Autodesk Fusion 360 part; units mm, degrees
(part 2 of 3)
  dimension "d109" = 3.1
  dimension "d110" = 3.1
  dimension "d111" = 3.1
  dimension "d112" = 3.1
  constraint parallel L339 L340
  constraint parallel L341 L342
  constraint tangent A29 L348
  constraint perpendicular L59 L347
  constraint perpendicular L59 L349
  constraint parallel L347 L348
  constraint parallel L10 L349
  constraint tangent A344 L353
  constraint tangent A347 L353
  constraint tangent L352 A347
  constraint tangent A344 L350
  constraint tangent A346 L352
  constraint tangent L350 A345
  constraint tangent L351 A346
  constraint tangent A345 L351
  constraint coincident P12 A348.centre
  constraint coincident P13 A349.centre
  constraint coincident P0 A350.centre
  constraint coincident P1 A351.centre
  constraint coincident P2 A352.centre
  constraint coincident P3 A353.centre
  constraint coincident P4 A354.centre
  constraint coincident P5 A355.centre
  constraint coincident P6 A356.centre
  constraint coincident P7 A357.centre
  constraint coincident P8 A358.centre
  constraint coincident P9 A359.centre
  constraint coincident P10 A360.centre
  constraint coincident P11 A361.centre
  constraint tangent L344 A341
  constraint tangent L343 A343
  constraint tangent L345 A342
  constraint tangent A341 L345
  constraint tangent L343 A340
  constraint tangent A340 L344
  constraint tangent A342 L346
  constraint tangent L346 A343
  measures "d99" diameter of A348
  measures "d100" diameter of A349
  measures "d101" diameter of A350
  measures "d102" diameter of A351
  measures "d103" diameter of A352
  measures "d104" diameter of A353
  measures "d105" diameter of A354
  measures "d106" diameter of A355
  measures "d107" diameter of A356
  measures "d108" diameter of A357
  measures "d109" diameter of A358
  measures "d110" diameter of A359
  measures "d111" diameter of A360
  measures "d112" diameter of A361
ref_plane "WorkPlane1" through (183.3563, -53.8188, -3) normal (0, 0, 1) x (1, 0, 0)
sketch "Sketch2" plane through (183.3563, -53.8188, -3) normal (0, 0, 1) x (1, 0, 0)
  line L0 (180.9997, -53.2885) -> (-181.0002, -53.2885)
  arc A0 (-185.0002, -49.2885) -> (-181.0002, -53.2885) centre (-181.0002, -49.2885) ccw
  line L1 (-185.0002, -49.2885) -> (-185.0002, 48.7115)
  arc A1 (-181.0002, 52.7115) -> (-185.0002, 48.7115) centre (-181.0002, 48.7115) ccw
  line L2 (-181.0002, 52.7115) -> (-28.9625, 52.7115)
  line L3 (-28.9625, 52.7115) -> (-28.9625, 55.9115)
  line L4 (-13.9625, 55.9115) -> (-13.9625, 52.7115)
  line L5 (-13.9625, 52.7115) -> (180.9997, 52.7115)
  arc A2 (184.9997, 48.7115) -> (180.9997, 52.7115) centre (180.9997, 48.7115) ccw
  line L6 (184.9997, 48.7115) -> (184.9997, -49.2885)
  arc A3 (180.9997, -53.2885) -> (184.9997, -49.2885) centre (180.9997, -49.2885) ccw
  line L7 (-13.9625, 55.9115) -> (-13.9625, 59.7113)
  line L8 (-28.9625, 55.9115) -> (-28.9625, 59.7113)
  arc A4 (196.0613, 54.7113) -> (188.0613, 62.7113) centre (188.0613, 54.7113) ccw
  line L9 (-13.9625, 62.7113) -> (188.0613, 62.7113)
  line L10 (-188.0613, 62.7113) -> (-28.9625, 62.7113)
  arc A5 (-188.0613, 62.7113) -> (-196.0613, 54.7113) centre (-188.0613, 54.7113) ccw
  line L11 (-196.0613, -54.7113) -> (-196.0613, 54.7113)
  arc A6 (-196.0613, -54.7113) -> (-188.0613, -62.7112) centre (-188.0613, -54.7113) ccw
  line L12 (188.0613, -62.7112) -> (-188.0613, -62.7112)
  arc A7 (188.0613, -62.7112) -> (196.0613, -54.7113) centre (188.0613, -54.7113) ccw
  line L13 (196.0612, 54.7113) -> (196.0612, -54.7113)
  line L14 (-28.9625, 59.7113) -> (-28.9625, 62.7113)
  line L15 (-13.9625, 59.7113) -> (-13.9625, 62.7113)
  line L16 (-61.8591, 54.9113) -> (-60.5312, 57.2113)
  line L17 (-60.5312, 57.2113) -> (-61.8591, 59.5113)
  line L18 (-61.8591, 59.5113) -> (-64.5149, 59.5113)
  line L19 (-64.5149, 59.5113) -> (-65.8428, 57.2113)
  line L20 (-65.8428, 57.2113) -> (-64.5149, 54.9113)
  line L21 (-64.5149, 54.9113) -> (-61.8591, 54.9113)
  line L22 (-125.0463, 54.9113) -> (-123.7184, 57.2113)
  line L23 (-123.7184, 57.2113) -> (-125.0463, 59.5113)
  line L24 (-125.0463, 59.5113) -> (-127.7022, 59.5113)
  line L25 (-127.7022, 59.5113) -> (-129.0301, 57.2113)
  line L26 (-129.0301, 57.2113) -> (-127.7022, 54.9113)
  line L27 (-127.7022, 54.9113) -> (-125.0463, 54.9113)
  line L28 (-188.2613, 29.4334) -> (-190.5613, 30.7613)
  line L29 (-190.5613, 30.7613) -> (-192.8613, 29.4334)
  line L30 (-192.8613, 29.4334) -> (-192.8613, 26.7776)
  line L31 (-192.8613, 26.7776) -> (-190.5613, 25.4497)
  line L32 (-190.5613, 25.4497) -> (-188.2613, 26.7776)
  line L33 (-188.2613, 26.7776) -> (-188.2613, 29.4334)
  line L34 (-188.2613, -26.7776) -> (-190.5613, -25.4497)
  line L35 (-190.5613, -25.4497) -> (-192.8613, -26.7776)
  line L36 (-192.8613, -26.7776) -> (-192.8613, -29.4334)
  line L37 (-192.8613, -29.4334) -> (-190.5613, -30.7613)
  line L38 (-190.5613, -30.7613) -> (-188.2613, -29.4334)
  line L39 (-188.2613, -29.4334) -> (-188.2613, -26.7776)
  line L40 (-127.7022, -54.9112) -> (-129.0301, -57.2112)
  line L41 (-129.0301, -57.2112) -> (-127.7022, -59.5112)
  line L42 (-127.7022, -59.5112) -> (-125.0463, -59.5112)
  line L43 (-125.0463, -59.5112) -> (-123.7184, -57.2112)
  line L44 (-123.7184, -57.2112) -> (-125.0463, -54.9112)
  line L45 (-125.0463, -54.9112) -> (-127.7022, -54.9112)
  line L46 (-64.5149, -54.9112) -> (-65.8428, -57.2112)
  line L47 (-65.8428, -57.2112) -> (-64.5149, -59.5112)
  line L48 (-64.5149, -59.5112) -> (-61.8591, -59.5112)
  line L49 (-61.8591, -59.5112) -> (-60.5312, -57.2112)
  line L50 (-60.5312, -57.2112) -> (-61.8591, -54.9112)
  line L51 (-61.8591, -54.9112) -> (-64.5149, -54.9112)
  line L52 (-1.3282, -54.9114) -> (-2.6558, -57.2116)
  line L53 (-2.6558, -57.2116) -> (-1.3276, -59.5114)
  line L54 (-1.3276, -59.5114) -> (1.3282, -59.5111)
  line L55 (1.3282, -59.5111) -> (2.6558, -57.2109)
  line L56 (2.6558, -57.2109) -> (1.3276, -54.9111)
  line L57 (1.3276, -54.9111) -> (-1.3282, -54.9114)
  line L58 (61.8591, -54.9112) -> (60.5312, -57.2112)
  line L59 (60.5312, -57.2112) -> (61.8591, -59.5112)
  line L60 (61.8591, -59.5112) -> (64.5149, -59.5112)
  line L61 (64.5149, -59.5112) -> (65.8428, -57.2112)
  line L62 (65.8428, -57.2112) -> (64.5149, -54.9112)
  line L63 (64.5149, -54.9112) -> (61.8591, -54.9112)
  line L64 (125.0463, -54.9112) -> (123.7184, -57.2112)
  line L65 (123.7184, -57.2112) -> (125.0463, -59.5112)
  line L66 (125.0463, -59.5112) -> (127.7022, -59.5112)
  line L67 (127.7022, -59.5112) -> (129.0301, -57.2112)
  line L68 (129.0301, -57.2112) -> (127.7022, -54.9112)
  line L69 (127.7022, -54.9112) -> (125.0463, -54.9112)
  line L70 (188.2612, -29.4334) -> (190.5612, -30.7613)
  line L71 (190.5612, -30.7613) -> (192.8612, -29.4334)
  line L72 (192.8612, -29.4334) -> (192.8612, -26.7776)
  line L73 (192.8612, -26.7776) -> (190.5612, -25.4497)
  line L74 (190.5612, -25.4497) -> (188.2612, -26.7776)
  line L75 (188.2612, -26.7776) -> (188.2612, -29.4334)
  line L76 (188.2612, 26.7776) -> (190.5612, 25.4497)
  line L77 (190.5612, 25.4497) -> (192.8612, 26.7776)
  line L78 (192.8612, 26.7776) -> (192.8612, 29.4334)
  line L79 (192.8612, 29.4334) -> (190.5612, 30.7613)
  line L80 (190.5612, 30.7613) -> (188.2612, 29.4334)
  line L81 (188.2612, 29.4334) -> (188.2612, 26.7776)
  line L82 (127.7022, 54.9113) -> (129.0301, 57.2113)
  line L83 (129.0301, 57.2113) -> (127.7022, 59.5113)
  line L84 (127.7022, 59.5113) -> (125.0463, 59.5113)
  line L85 (125.0463, 59.5113) -> (123.7184, 57.2113)
  line L86 (123.7184, 57.2113) -> (125.0463, 54.9113)
  line L87 (125.0463, 54.9113) -> (127.7022, 54.9113)
  line L88 (64.5149, 54.9113) -> (65.8428, 57.2113)
  line L89 (65.8428, 57.2113) -> (64.5149, 59.5113)
  line L90 (64.5149, 59.5113) -> (61.8591, 59.5113)
  line L91 (61.8591, 59.5113) -> (60.5312, 57.2113)
  line L92 (60.5312, 57.2113) -> (61.8591, 54.9113)
  line L93 (61.8591, 54.9113) -> (64.5149, 54.9113)
  line L94 (1.3279, 54.9113) -> (2.6558, 57.2113)
  line L95 (2.6558, 57.2113) -> (1.3279, 59.5113)
  line L96 (1.3279, 59.5113) -> (-1.3279, 59.5113)
  line L97 (-1.3279, 59.5113) -> (-2.6558, 57.2113)
  line L98 (-2.6558, 57.2113) -> (-1.3279, 54.9113)
  line L99 (-1.3279, 54.9113) -> (1.3279, 54.9113)
  point P0 (-126.3743, 57.2113)
  point P1 (-190.5613, 28.1055)
  point P2 (-190.5613, -28.1055)
  point P3 (-126.3743, -57.2112)
  point P4 (-63.187, -57.2112)
  point P5 (0, -57.2112)
  point P6 (63.187, -57.2112)
  point P7 (126.3742, -57.2112)
  point P8 (190.5612, -28.1055)
  point P9 (190.5612, 28.1055)
  point P10 (126.3742, 57.2113)
  point P11 (63.187, 57.2113)
  point P12 (0, 57.2113)
  point P13 (-63.187, 57.2113)
  point P14 (0, 57.2113)
  point P15 (-63.187, 57.2113)
  point P16 (-126.3743, 57.2113)
  point P17 (-190.5613, 28.1055)
  point P18 (-190.5613, -28.1055)
  point P19 (-126.3743, -57.2112)
  point P20 (-63.187, -57.2112)
  point P21 (0, -57.2112)
  point P22 (63.187, -57.2112)
  point P23 (126.3742, -57.2112)
  point P24 (190.5612, -28.1055)
  point P25 (190.5612, 28.1055)
  point P26 (126.3742, 57.2113)
  point P27 (63.187, 57.2113)
  point P28 (-63.187, 57.2113)
  point P29 (-126.3743, 57.2113)
  point P30 (-190.5613, 28.1055)
  point P31 (-190.5613, -28.1055)
  point P32 (-126.3743, -57.2112)
  point P33 (-63.187, -57.2112)
  point P34 (0, -57.2112)
  point P35 (63.187, -57.2112)
  point P36 (126.3742, -57.2112)
  point P37 (190.5612, -28.1055)
  point P38 (190.5612, 28.1055)
  point P39 (126.3742, 57.2113)
  point P40 (63.187, 57.2113)
  point P41 (0, 57.2113)
  dimension "d113" = 2.3
  dimension "d114" = 2.3
  dimension "d115" = 2.3
  dimension "d116" = 2.3
  dimension "d117" = 2.3
  dimension "d118" = 2.3
  dimension "d119" = 2.3
  dimension "d120" = 2.3
  dimension "d121" = 2.3
  dimension "d122" = 2.3
  dimension "d123" = 2.3
  dimension "d124" = 2.3
  dimension "d125" = 2.3
  dimension "d126" = 2.3
  constraint tangent L1 A1
  constraint tangent L0 A3
  constraint tangent L0 A0
  constraint tangent A0 L1
  constraint tangent A1 L2
  constraint tangent L5 A2
  constraint tangent A2 L6
  constraint tangent L6 A3
  constraint perpendicular L10 L14
  constraint perpendicular L9 L15
  constraint tangent A4 L13
  constraint tangent A4 L9
  constraint tangent L10 A5
  constraint tangent A5 L11
  constraint tangent L11 A6
  constraint tangent A6 L12
  constraint tangent L12 A7
  constraint tangent A7 L13
  constraint coincident P41 P14
  constraint coincident P28 P15
  constraint coincident P29 P16
  constraint coincident P30 P17
  constraint coincident P31 P18
  constraint coincident P32 P19
  constraint coincident P33 P20
  constraint coincident P34 P21
  constraint coincident P35 P22
  constraint coincident P36 P23
  constraint coincident P37 P24
  constraint coincident P38 P25
  constraint coincident P39 P26
  constraint coincident P40 P27
  measures "d113" distance of P28 L21
  measures "d114" distance of P29 L27
  measures "d115" distance of P30 L33
  measures "d116" distance of P31 L39
  measures "d117" distance of P32 L45
  measures "d118" distance of P33 L51
  measures "d119" distance of P34 L57
  measures "d120" distance of P35 L63
  measures "d121" distance of P36 L69
  measures "d122" distance of P37 L75
  measures "d123" distance of P38 L81
  measures "d124" distance of P39 L87
  measures "d125" distance of P40 L93
  measures "d126" distance of P41 L99
ref_plane "WorkPlane2" through (183.3562, -53.8188, -9) normal (0, 0, 1) x (1, 0, 0)
ref_plane "WorkPlane3" through (183.3562, -53.8188, -9) normal (0, 0, 1) x (1, 0, 0)
sketch "Sketch4" plane through (183.3562, -53.8188, -9) normal (0, 0, 1) x (1, 0, 0)
  line L0 (-188.0613, 62.7113) -> (188.0613, 62.7113)
  arc A0 (-188.0613, 62.7113) -> (-196.0613, 54.7113) centre (-188.0613, 54.7113) ccw
  line L1 (-196.0613, -54.7113) -> (-196.0613, 54.7113)
  circle A1 centre (-190.5613, 28.1055) radius 1.55
  circle A2 centre (-190.5613, -28.1055) radius 1.55
  circle A3 centre (-126.3742, 57.2113) radius 1.55
  arc A4 (-196.0613, -54.7113) -> (-188.0613, -62.7113) centre (-188.0613, -54.7113) ccw
  line L2 (188.0613, -62.7113) -> (-188.0613, -62.7112)
  circle A5 centre (-126.3742, -57.2113) radius 1.55
  circle A6 centre (-63.187, -57.2113) radius 1.55
  circle A7 centre (-63.187, 57.2113) radius 1.55
  circle A8 centre (0, 57.2113) radius 1.55
  circle A9 centre (0, -57.2113) radius 1.55
  circle A10 centre (63.187, -57.2113) radius 1.55
  circle A11 centre (126.3742, -57.2113) radius 1.55
  circle A12 centre (63.187, 57.2113) radius 1.55
  circle A13 centre (126.3742, 57.2113) radius 1.55
  arc A14 (196.0612, 54.7113) -> (188.0613, 62.7112) centre (188.0613, 54.7113) ccw
  line L3 (196.0612, 54.7113) -> (196.0613, -54.7113)
  circle A15 centre (190.5613, 28.1055) radius 1.55
  circle A16 centre (190.5613, -28.1055) radius 1.55
  arc A17 (188.0613, -62.7113) -> (196.0613, -54.7113) centre (188.0613, -54.7113) ccw
  point P0 (0, -57.2113)
  point P1 (0, 57.2113)
  point P2 (126.3742, 57.2113)
extrude "Extrude8" add sketch "Frogdor Top Plate" against normal blind 3 makes body 1
extrude "Extrude9" add sketch "Sketch2" against normal blind 6 separate body makes body 2
extrude "Extrude10" add sketch "Sketch4" against normal blind 3 separate body makes body 3
sketch "Sketch5" plane through (0, 0, 0) normal (0, 0, 1) x (-1, 0, 0)
  arc A0 (-351.1875, 6.3375) -> (-350.1875, 7.3375) centre (-351.1875, 7.3375) ccw
  line L0 (-351.1875, 6.3375) -> (-363.1875, 6.3375)
  arc A1 (-364.1875, 7.3375) -> (-363.1875, 6.3375) centre (-363.1875, 7.3375) ccw
  line L1 (-364.1875, 7.3375) -> (-364.1875, 19.3375)
  arc A2 (-363.1875, 20.3375) -> (-364.1875, 19.3375) centre (-363.1875, 19.3375) ccw
  line L2 (-363.1875, 20.3375) -> (-351.1875, 20.3375)
  arc A3 (-350.1875, 19.3375) -> (-351.1875, 20.3375) centre (-351.1875, 19.3375) ccw
  line L3 (-350.1875, 19.3375) -> (-350.1875, 7.3375)
  arc A4 (-187.975, 26.3875) -> (-186.975, 25.3875) centre (-186.975, 26.3875) ccw
  line L4 (-187.975, 26.3875) -> (-187.975, 38.3875)
  arc A5 (-186.975, 39.3875) -> (-187.975, 38.3875) centre (-186.975, 38.3875) ccw
  line L5 (-186.975, 39.3875) -> (-174.975, 39.3875)
  arc A6 (-173.975, 38.3875) -> (-174.975, 39.3875) centre (-174.975, 38.3875) ccw
  line L6 (-173.975, 38.3875) -> (-173.975, 26.3875)
  arc A7 (-174.975, 25.3875) -> (-173.975, 26.3875) centre (-174.975, 26.3875) ccw
  line L7 (-174.975, 25.3875) -> (-186.975, 25.3875)
  arc A8 (-270.225, 25.3875) -> (-269.225, 26.3875) centre (-270.225, 26.3875) ccw
  line L8 (-270.225, 25.3875) -> (-282.225, 25.3875)
  arc A9 (-283.225, 26.3875) -> (-282.225, 25.3875) centre (-282.225, 26.3875) ccw
  line L9 (-283.225, 26.3875) -> (-283.225, 38.3875)
  arc A10 (-282.225, 39.3875) -> (-283.225, 38.3875) centre (-282.225, 38.3875) ccw
  line L10 (-282.225, 39.3875) -> (-270.225, 39.3875)
  arc A11 (-269.225, 38.3875) -> (-270.225, 39.3875) centre (-270.225, 38.3875) ccw
  line L11 (-269.225, 38.3875) -> (-269.225, 26.3875)
  arc A12 (-313.0875, 25.3875) -> (-312.0875, 26.3875) centre (-313.0875, 26.3875) ccw
  line L12 (-313.0875, 25.3875) -> (-325.0875, 25.3875)
  arc A13 (-326.0875, 26.3875) -> (-325.0875, 25.3875) centre (-325.0875, 26.3875) ccw
  line L13 (-326.0875, 26.3875) -> (-326.0875, 38.3875)
  arc A14 (-325.0875, 39.3875) -> (-326.0875, 38.3875) centre (-325.0875, 38.3875) ccw
  line L14 (-325.0875, 39.3875) -> (-313.0875, 39.3875)
  arc A15 (-312.0875, 38.3875) -> (-313.0875, 39.3875) centre (-313.0875, 38.3875) ccw
  line L15 (-312.0875, 38.3875) -> (-312.0875, 26.3875)
  arc A16 (-305.9438, 44.4375) -> (-304.9438, 45.4375) centre (-305.9438, 45.4375) ccw
  line L16 (-305.9438, 44.4375) -> (-317.9438, 44.4375)
  arc A17 (-318.9438, 45.4375) -> (-317.9438, 44.4375) centre (-317.9438, 45.4375) ccw
  line L17 (-318.9438, 45.4375) -> (-318.9438, 57.4375)
  arc A18 (-317.9438, 58.4375) -> (-318.9438, 57.4375) centre (-317.9438, 57.4375) ccw
  line L18 (-317.9438, 58.4375) -> (-305.9438, 58.4375)
  arc A19 (-304.9438, 57.4375) -> (-305.9438, 58.4375) centre (-305.9438, 57.4375) ccw
  line L19 (-304.9438, 57.4375) -> (-304.9438, 45.4375)
  arc A20 (-217.8375, 44.4375) -> (-216.8375, 45.4375) centre (-217.8375, 45.4375) ccw
  line L20 (-217.8375, 44.4375) -> (-229.8375, 44.4375)
  arc A21 (-230.8375, 45.4375) -> (-229.8375, 44.4375) centre (-229.8375, 45.4375) ccw
  line L21 (-230.8375, 45.4375) -> (-230.8375, 57.4375)
  arc A22 (-229.8375, 58.4375) -> (-230.8375, 57.4375) centre (-229.8375, 57.4375) ccw
  line L22 (-229.8375, 58.4375) -> (-217.8375, 58.4375)
  arc A23 (-216.8375, 57.4375) -> (-217.8375, 58.4375) centre (-217.8375, 57.4375) ccw
  line L23 (-216.8375, 57.4375) -> (-216.8375, 45.4375)
  arc A24 (-122.5875, 44.4375) -> (-121.5875, 45.4375) centre (-122.5875, 45.4375) ccw
  line L24 (-122.5875, 44.4375) -> (-134.5875, 44.4375)
  arc A25 (-135.5875, 45.4375) -> (-134.5875, 44.4375) centre (-134.5875, 45.4375) ccw
  line L25 (-135.5875, 45.4375) -> (-135.5875, 57.4375)
  arc A26 (-134.5875, 58.4375) -> (-135.5875, 57.4375) centre (-134.5875, 57.4375) ccw
  line L26 (-134.5875, 58.4375) -> (-122.5875, 58.4375)
  arc A27 (-121.5875, 57.4375) -> (-122.5875, 58.4375) centre (-122.5875, 57.4375) ccw
  line L27 (-121.5875, 57.4375) -> (-121.5875, 45.4375)
  arc A28 (-236.8875, 44.4375) -> (-235.8875, 45.4375) centre (-236.8875, 45.4375) ccw
  line L28 (-236.8875, 44.4375) -> (-248.8875, 44.4375)
  arc A29 (-249.8875, 45.4375) -> (-248.8875, 44.4375) centre (-248.8875, 45.4375) ccw
  line L29 (-249.8875, 45.4375) -> (-249.8875, 57.4375)
  arc A30 (-248.8875, 58.4375) -> (-249.8875, 57.4375) centre (-248.8875, 57.4375) ccw
  line L30 (-248.8875, 58.4375) -> (-236.8875, 58.4375)
  arc A31 (-235.8875, 57.4375) -> (-236.8875, 58.4375) centre (-236.8875, 57.4375) ccw
  line L31 (-235.8875, 57.4375) -> (-235.8875, 45.4375)
  arc A32 (-297.5057, 45.4375) -> (-296.5057, 46.4375) centre (-297.5057, 46.4375) ccw
  line L32 (-297.5057, 45.4375) -> (-302.5057, 45.4375)
  arc A33 (-303.5057, 46.4375) -> (-302.5057, 45.4375) centre (-302.5057, 46.4375) ccw
  line L33 (-303.5057, 46.4375) -> (-303.5057, 59.4375)
  arc A34 (-302.5057, 60.4375) -> (-303.5058, 59.4375) centre (-302.5058, 59.4375) ccw
  line L34 (-302.5057, 60.4375) -> (-297.5057, 60.4375)
  arc A35 (-296.5057, 59.4375) -> (-297.5057, 60.4375) centre (-297.5057, 59.4375) ccw
  line L35 (-296.5057, 59.4375) -> (-296.5057, 46.4375)
  arc A36 (-117.825, 25.3875) -> (-116.825, 26.3875) centre (-117.825, 26.3875) ccw
  line L36 (-117.825, 25.3875) -> (-129.825, 25.3875)
  arc A37 (-130.825, 26.3875) -> (-129.825, 25.3875) centre (-129.825, 26.3875) ccw
  line L37 (-130.825, 26.3875) -> (-130.825, 38.3875)
  arc A38 (-129.825, 39.3875) -> (-130.825, 38.3875) centre (-129.825, 38.3875) ccw
  line L38 (-129.825, 39.3875) -> (-117.825, 39.3875)
  arc A39 (-116.825, 38.3875) -> (-117.825, 39.3875) centre (-117.825, 38.3875) ccw
  line L39 (-116.825, 38.3875) -> (-116.825, 26.3875)
  arc A40 (-3.525, 25.3875) -> (-2.525, 26.3875) centre (-3.525, 26.3875) ccw
  line L40 (-3.525, 25.3875) -> (-15.525, 25.3875)
  arc A41 (-16.525, 26.3875) -> (-15.525, 25.3875) centre (-15.525, 26.3875) ccw
  line L41 (-16.525, 26.3875) -> (-16.525, 38.3875)
  arc A42 (-15.525, 39.3875) -> (-16.525, 38.3875) centre (-15.525, 38.3875) ccw
  line L42 (-15.525, 39.3875) -> (-3.525, 39.3875)
  arc A43 (-2.525, 38.3875) -> (-3.525, 39.3875) centre (-3.525, 38.3875) ccw
  line L43 (-2.525, 38.3875) -> (-2.525, 26.3875)
  line L44 (-83.4875, 57.4375) -> (-83.4875, 45.4375)
  arc A44 (-84.4875, 44.4375) -> (-83.4875, 45.4375) centre (-84.4875, 45.4375) ccw
  line L45 (-84.4875, 44.4375) -> (-96.4875, 44.4375)
  arc A45 (-97.4875, 45.4375) -> (-96.4875, 44.4375) centre (-96.4875, 45.4375) ccw
  line L46 (-97.4875, 45.4375) -> (-97.4875, 57.4375)
  arc A46 (-96.4875, 58.4375) -> (-97.4875, 57.4375) centre (-96.4875, 57.4375) ccw
  line L47 (-96.4875, 58.4375) -> (-84.4875, 58.4375)
  arc A47 (-83.4875, 57.4375) -> (-84.4875, 58.4375) centre (-84.4875, 57.4375) ccw
  arc A48 (-103.5375, 44.4375) -> (-102.5375, 45.4375) centre (-103.5375, 45.4375) ccw
  line L48 (-103.5375, 44.4375) -> (-115.5375, 44.4375)
  arc A49 (-116.5375, 45.4375) -> (-115.5375, 44.4375) centre (-115.5375, 45.4375) ccw
  line L49 (-116.5375, 45.4375) -> (-116.5375, 57.4375)
  arc A50 (-115.5375, 58.4375) -> (-116.5375, 57.4375) centre (-115.5375, 57.4375) ccw
  line L50 (-115.5375, 58.4375) -> (-103.5375, 58.4375)
  arc A51 (-102.5375, 57.4375) -> (-103.5375, 58.4375) centre (-103.5375, 57.4375) ccw
  line L51 (-102.5375, 57.4375) -> (-102.5375, 45.4375)
  arc A52 (-255.9375, 44.4375) -> (-254.9375, 45.4375) centre (-255.9375, 45.4375) ccw
  line L52 (-255.9375, 44.4375) -> (-267.9375, 44.4375)
  arc A53 (-268.9375, 45.4375) -> (-267.9375, 44.4375) centre (-267.9375, 45.4375) ccw
  line L53 (-268.9375, 45.4375) -> (-268.9375, 57.4375)
  arc A54 (-267.9375, 58.4375) -> (-268.9375, 57.4375) centre (-267.9375, 57.4375) ccw
  line L54 (-267.9375, 58.4375) -> (-255.9375, 58.4375)
  arc A55 (-254.9375, 57.4375) -> (-255.9375, 58.4375) centre (-255.9375, 57.4375) ccw
  line L55 (-254.9375, 57.4375) -> (-254.9375, 45.4375)
  arc A56 (-165.45, 6.3375) -> (-164.45, 7.3375) centre (-165.45, 7.3375) ccw
  line L56 (-165.45, 6.3375) -> (-177.45, 6.3375)
  arc A57 (-178.45, 7.3375) -> (-177.45, 6.3375) centre (-177.45, 7.3375) ccw
  line L57 (-178.45, 7.3375) -> (-178.45, 19.3375)
  arc A58 (-177.45, 20.3375) -> (-178.45, 19.3375) centre (-177.45, 19.3375) ccw
  line L58 (-177.45, 20.3375) -> (-165.45, 20.3375)
  arc A59 (-164.45, 19.3375) -> (-165.45, 20.3375) centre (-165.45, 19.3375) ccw
  line L59 (-164.45, 19.3375) -> (-164.45, 7.3375)
  arc A60 (-226.075, 26.3875) -> (-225.075, 25.3875) centre (-225.075, 26.3875) ccw
  line L60 (-226.075, 26.3875) -> (-226.075, 38.3875)
  arc A61 (-225.075, 39.3875) -> (-226.075, 38.3875) centre (-225.075, 38.3875) ccw
  line L61 (-225.075, 39.3875) -> (-213.075, 39.3875)
  arc A62 (-212.075, 38.3875) -> (-213.075, 39.3875) centre (-213.075, 38.3875) ccw
  line L62 (-212.075, 38.3875) -> (-212.075, 26.3875)
  arc A63 (-213.075, 25.3875) -> (-212.075, 26.3875) centre (-213.075, 26.3875) ccw
  line L63 (-213.075, 25.3875) -> (-225.075, 25.3875)
  arc A64 (-194.025, 25.3875) -> (-193.025, 26.3875) centre (-194.025, 26.3875) ccw
  line L64 (-194.025, 25.3875) -> (-206.025, 25.3875)
  arc A65 (-207.025, 26.3875) -> (-206.025, 25.3875) centre (-206.025, 26.3875) ccw
  line L65 (-207.025, 26.3875) -> (-207.025, 38.3875)
  arc A66 (-206.025, 39.3875) -> (-207.025, 38.3875) centre (-206.025, 38.3875) ccw
  line L66 (-206.025, 39.3875) -> (-194.025, 39.3875)
  arc A67 (-193.025, 38.3875) -> (-194.025, 39.3875) centre (-194.025, 38.3875) ccw
  line L67 (-193.025, 38.3875) -> (-193.025, 26.3875)
  arc A68 (-260.7, 6.3375) -> (-259.7, 7.3375) centre (-260.7, 7.3375) ccw
  line L68 (-260.7, 6.3375) -> (-272.7, 6.3375)
  arc A69 (-273.7, 7.3375) -> (-272.7, 6.3375) centre (-272.7, 7.3375) ccw
  line L69 (-273.7, 7.3375) -> (-273.7, 19.3375)
  arc A70 (-272.7, 20.3375) -> (-273.7, 19.3375) centre (-272.7, 19.3375) ccw
  line L70 (-272.7, 20.3375) -> (-260.7, 20.3375)
  arc A71 (-259.7, 19.3375) -> (-260.7, 20.3375) centre (-260.7, 19.3375) ccw
  line L71 (-259.7, 19.3375) -> (-259.7, 7.3375)
  arc A72 (-160.6875, 44.4375) -> (-159.6875, 45.4375) centre (-160.6875, 45.4375) ccw
  line L72 (-160.6875, 44.4375) -> (-172.6875, 44.4375)
  arc A73 (-173.6875, 45.4375) -> (-172.6875, 44.4375) centre (-172.6875, 45.4375) ccw
  line L73 (-173.6875, 45.4375) -> (-173.6875, 57.4375)
  arc A74 (-172.6875, 58.4375) -> (-173.6875, 57.4375) centre (-172.6875, 57.4375) ccw
  line L74 (-172.6875, 58.4375) -> (-160.6875, 58.4375)
  arc A75 (-159.6875, 57.4375) -> (-160.6875, 58.4375) centre (-160.6875, 57.4375) ccw
  line L75 (-159.6875, 57.4375) -> (-159.6875, 45.4375)
  arc A76 (-55.9125, 25.3875) -> (-54.9125, 26.3875) centre (-55.9125, 26.3875) ccw
  line L76 (-55.9125, 25.3875) -> (-67.9125, 25.3875)
  arc A77 (-68.9125, 26.3875) -> (-67.9125, 25.3875) centre (-67.9125, 26.3875) ccw
  line L77 (-68.9125, 26.3875) -> (-68.9125, 38.3875)
  arc A78 (-67.9125, 39.3875) -> (-68.9125, 38.3875) centre (-67.9125, 38.3875) ccw
  line L78 (-67.9125, 39.3875) -> (-55.9125, 39.3875)
  arc A79 (-54.9125, 38.3875) -> (-55.9125, 39.3875) centre (-55.9125, 38.3875) ccw
  line L79 (-54.9125, 38.3875) -> (-54.9125, 26.3875)
  arc A80 (-351.1875, 25.3875) -> (-350.1875, 26.3875) centre (-351.1875, 26.3875) ccw
  line L80 (-351.1875, 25.3875) -> (-363.1875, 25.3875)
  arc A81 (-364.1875, 26.3875) -> (-363.1875, 25.3875) centre (-363.1875, 26.3875) ccw
  line L81 (-364.1875, 26.3875) -> (-364.1875, 38.3875)
  arc A82 (-363.1875, 39.3875) -> (-364.1875, 38.3875) centre (-363.1875, 38.3875) ccw
  line L82 (-363.1875, 39.3875) -> (-351.1875, 39.3875)
  arc A83 (-350.1875, 38.3875) -> (-351.1875, 39.3875) centre (-351.1875, 38.3875) ccw
  line L83 (-350.1875, 38.3875) -> (-350.1875, 26.3875)
  arc A84 (-79.725, 25.3875) -> (-78.725, 26.3875) centre (-79.725, 26.3875) ccw
  line L84 (-79.725, 25.3875) -> (-91.725, 25.3875)
  arc A85 (-92.725, 26.3875) -> (-91.725, 25.3875) centre (-91.725, 26.3875) ccw
  line L85 (-92.725, 26.3875) -> (-92.725, 38.3875)
  arc A86 (-91.725, 39.3875) -> (-92.725, 38.3875) centre (-91.725, 38.3875) ccw
  line L86 (-91.725, 39.3875) -> (-79.725, 39.3875)
  arc A87 (-78.725, 38.3875) -> (-79.725, 39.3875) centre (-79.725, 38.3875) ccw
  line L87 (-78.725, 38.3875) -> (-78.725, 26.3875)
  arc A88 (-155.925, 25.3875) -> (-154.925, 26.3875) centre (-155.925, 26.3875) ccw
  line L88 (-155.925, 25.3875) -> (-167.925, 25.3875)
  arc A89 (-168.925, 26.3875) -> (-167.925, 25.3875) centre (-167.925, 26.3875) ccw
  line L89 (-168.925, 26.3875) -> (-168.925, 38.3875)
  arc A90 (-167.925, 39.3875) -> (-168.925, 38.3875) centre (-167.925, 38.3875) ccw
  line L90 (-167.925, 39.3875) -> (-155.925, 39.3875)
  arc A91 (-154.925, 38.3875) -> (-155.925, 39.3875) centre (-155.925, 38.3875) ccw
  line L91 (-154.925, 38.3875) -> (-154.925, 26.3875)
  arc A92 (-22.575, 44.4375) -> (-21.575, 45.4375) centre (-22.575, 45.4375) ccw
  line L92 (-22.575, 44.4375) -> (-34.575, 44.4375)
  arc A93 (-35.575, 45.4375) -> (-34.575, 44.4375) centre (-34.575, 45.4375) ccw
  line L93 (-35.575, 45.4375) -> (-35.575, 57.4375)
  arc A94 (-34.575, 58.4375) -> (-35.575, 57.4375) centre (-34.575, 57.4375) ccw
  line L94 (-34.575, 58.4375) -> (-22.575, 58.4375)
  arc A95 (-21.575, 57.4375) -> (-22.575, 58.4375) centre (-22.575, 57.4375) ccw
  line L95 (-21.575, 57.4375) -> (-21.575, 45.4375)
  arc A96 (-289.275, 25.3875) -> (-288.275, 26.3875) centre (-289.275, 26.3875) ccw
  line L96 (-289.275, 25.3875) -> (-301.275, 25.3875)
  arc A97 (-302.275, 26.3875) -> (-301.275, 25.3875) centre (-301.275, 26.3875) ccw
  line L97 (-302.275, 26.3875) -> (-302.275, 38.3875)
  arc A98 (-301.275, 39.3875) -> (-302.275, 38.3875) centre (-301.275, 38.3875) ccw
  line L98 (-301.275, 39.3875) -> (-289.275, 39.3875)
  arc A99 (-288.275, 38.3875) -> (-289.275, 39.3875) centre (-289.275, 38.3875) ccw
  line L99 (-288.275, 38.3875) -> (-288.275, 26.3875)
  arc A100 (-179.7375, 44.4375) -> (-178.7375, 45.4375) centre (-179.7375, 45.4375) ccw
  line L100 (-179.7375, 44.4375) -> (-191.7375, 44.4375)
  arc A101 (-192.7375, 45.4375) -> (-191.7375, 44.4375) centre (-191.7375, 45.4375) ccw
  line L101 (-192.7375, 45.4375) -> (-192.7375, 57.4375)
  arc A102 (-191.7375, 58.4375) -> (-192.7375, 57.4375) centre (-191.7375, 57.4375) ccw
  line L102 (-191.7375, 58.4375) -> (-179.7375, 58.4375)
  arc A103 (-178.7375, 57.4375) -> (-179.7375, 58.4375) centre (-179.7375, 57.4375) ccw
  line L103 (-178.7375, 57.4375) -> (-178.7375, 45.4375)
  arc A104 (-136.875, 25.3875) -> (-135.875, 26.3875) centre (-136.875, 26.3875) ccw
  line L104 (-136.875, 25.3875) -> (-148.875, 25.3875)
  arc A105 (-149.875, 26.3875) -> (-148.875, 25.3875) centre (-148.875, 26.3875) ccw
  line L105 (-149.875, 26.3875) -> (-149.875, 38.3875)
  arc A106 (-148.875, 39.3875) -> (-149.875, 38.3875) centre (-148.875, 38.3875) ccw
  line L106 (-148.875, 39.3875) -> (-136.875, 39.3875)
  arc A107 (-135.875, 38.3875) -> (-136.875, 39.3875) centre (-136.875, 38.3875) ccw
  line L107 (-135.875, 38.3875) -> (-135.875, 26.3875)
  arc A108 (-22.575, 25.3875) -> (-21.575, 26.3875) centre (-22.575, 26.3875) ccw
  line L108 (-22.575, 25.3875) -> (-34.575, 25.3875)
  arc A109 (-35.575, 26.3875) -> (-34.575, 25.3875) centre (-34.575, 26.3875) ccw
  line L109 (-35.575, 26.3875) -> (-35.575, 38.3875)
  arc A110 (-34.575, 39.3875) -> (-35.575, 38.3875) centre (-34.575, 38.3875) ccw
  line L110 (-34.575, 39.3875) -> (-22.575, 39.3875)
  arc A111 (-21.575, 38.3875) -> (-22.575, 39.3875) centre (-22.575, 38.3875) ccw
  line L111 (-21.575, 38.3875) -> (-21.575, 26.3875)
  arc A112 (-251.175, 25.3875) -> (-250.175, 26.3875) centre (-251.175, 26.3875) ccw
  line L112 (-251.175, 25.3875) -> (-263.175, 25.3875)
  arc A113 (-264.175, 26.3875) -> (-263.175, 25.3875) centre (-263.175, 26.3875) ccw
  line L113 (-264.175, 26.3875) -> (-264.175, 38.3875)
  arc A114 (-263.175, 39.3875) -> (-264.175, 38.3875) centre (-263.175, 38.3875) ccw
  line L114 (-263.175, 39.3875) -> (-251.175, 39.3875)
  arc A115 (-250.175, 38.3875) -> (-251.175, 39.3875) centre (-251.175, 38.3875) ccw
  line L115 (-250.175, 38.3875) -> (-250.175, 26.3875)
  arc A116 (-279.75, 6.3375) -> (-278.75, 7.3375) centre (-279.75, 7.3375) ccw
  line L116 (-279.75, 6.3375) -> (-291.75, 6.3375)
  arc A117 (-292.75, 7.3375) -> (-291.75, 6.3375) centre (-291.75, 7.3375) ccw
  line L117 (-292.75, 7.3375) -> (-292.75, 19.3375)
  arc A118 (-291.75, 20.3375) -> (-292.75, 19.3375) centre (-291.75, 19.3375) ccw
  line L118 (-291.75, 20.3375) -> (-279.75, 20.3375)
  arc A119 (-278.75, 19.3375) -> (-279.75, 20.3375) centre (-279.75, 19.3375) ccw
  line L119 (-278.75, 19.3375) -> (-278.75, 7.3375)
  arc A120 (-3.525, 44.4375) -> (-2.525, 45.4375) centre (-3.525, 45.4375) ccw
  line L120 (-3.525, 44.4375) -> (-15.525, 44.4375)
  arc A121 (-16.525, 45.4375) -> (-15.525, 44.4375) centre (-15.525, 45.4375) ccw
  line L121 (-16.525, 45.4375) -> (-16.525, 57.4375)
  arc A122 (-15.525, 58.4375) -> (-16.525, 57.4375) centre (-15.525, 57.4375) ccw
  line L122 (-15.525, 58.4375) -> (-3.525, 58.4375)
  arc A123 (-2.525, 57.4375) -> (-3.525, 58.4375) centre (-3.525, 57.4375) ccw
  line L123 (-2.525, 57.4375) -> (-2.525, 45.4375)
  arc A124 (-141.6375, 44.4375) -> (-140.6375, 45.4375) centre (-141.6375, 45.4375) ccw
  line L124 (-141.6375, 44.4375) -> (-153.6375, 44.4375)
  arc A125 (-154.6375, 45.4375) -> (-153.6375, 44.4375) centre (-153.6375, 45.4375) ccw
  line L125 (-154.6375, 45.4375) -> (-154.6375, 57.4375)
  arc A126 (-153.6375, 58.4375) -> (-154.6375, 57.4375) centre (-153.6375, 57.4375) ccw
  line L126 (-153.6375, 58.4375) -> (-141.6375, 58.4375)
  arc A127 (-140.6375, 57.4375) -> (-141.6375, 58.4375) centre (-141.6375, 57.4375) ccw
  line L127 (-140.6375, 57.4375) -> (-140.6375, 45.4375)
  arc A128 (-98.775, 25.3875) -> (-97.775, 26.3875) centre (-98.775, 26.3875) ccw
  line L128 (-98.775, 25.3875) -> (-110.775, 25.3875)
  arc A129 (-111.775, 26.3875) -> (-110.775, 25.3875) centre (-110.775, 26.3875) ccw
  line L129 (-111.775, 26.3875) -> (-111.775, 38.3875)
  arc A130 (-110.775, 39.3875) -> (-111.775, 38.3875) centre (-110.775, 38.3875) ccw
  line L130 (-110.775, 39.3875) -> (-98.775, 39.3875)
  arc A131 (-97.775, 38.3875) -> (-98.775, 39.3875) centre (-98.775, 38.3875) ccw
  line L131 (-97.775, 38.3875) -> (-97.775, 26.3875)
  arc A132 (-232.125, 25.3875) -> (-231.125, 26.3875) centre (-232.125, 26.3875) ccw
  line L132 (-232.125, 25.3875) -> (-244.125, 25.3875)
  arc A133 (-245.125, 26.3875) -> (-244.125, 25.3875) centre (-244.125, 26.3875) ccw
  line L133 (-245.125, 26.3875) -> (-245.125, 38.3875)
  arc A134 (-244.125, 39.3875) -> (-245.125, 38.3875) centre (-244.125, 38.3875) ccw
  line L134 (-244.125, 39.3875) -> (-232.125, 39.3875)
  arc A135 (-231.125, 38.3875) -> (-232.125, 39.3875) centre (-232.125, 38.3875) ccw
  line L135 (-231.125, 38.3875) -> (-231.125, 26.3875)
  circle A136 centre (7.205, 25.7132) radius 1.55
  arc A137 (-274.9875, 44.4375) -> (-273.9875, 45.4375) centre (-274.9875, 45.4375) ccw
  line L136 (-274.9875, 44.4375) -> (-286.9875, 44.4375)
  arc A138 (-287.9875, 45.4375) -> (-286.9875, 44.4375) centre (-286.9875, 45.4375) ccw
  line L137 (-287.9875, 45.4375) -> (-287.9875, 57.4375)
  arc A139 (-286.9875, 58.4375) -> (-287.9875, 57.4375) centre (-286.9875, 57.4375) ccw
  line L138 (-286.9875, 58.4375) -> (-274.9875, 58.4375)
  arc A140 (-273.9875, 57.4375) -> (-274.9875, 58.4375) centre (-274.9875, 57.4375) ccw
  line L139 (-273.9875, 57.4375) -> (-273.9875, 45.4375)
  circle A141 centre (7.205, 81.9243) radius 1.55
  circle A142 centre (-56.982, 111.03) radius 1.55
  circle A143 centre (-120.1693, 111.03) radius 1.55
  circle A144 centre (-183.3563, 111.03) radius 1.55
  circle A145 centre (-246.5433, 111.03) radius 1.55
  circle A146 centre (-309.7305, 111.03) radius 1.55
  circle A147 centre (-373.9175, 81.9243) radius 1.55
  circle A148 centre (-373.9175, 25.7132) radius 1.55
  circle A149 centre (-309.7305, -3.3925) radius 1.55
  circle A150 centre (-246.5433, -3.3925) radius 1.55
  circle A151 centre (-183.3563, -3.3925) radius 1.55
  circle A152 centre (-120.1693, -3.3925) radius 1.55
  circle A153 centre (-56.982, -3.3925) radius 1.55
  arc A154 (-221.3313, 83.51) -> (-220.2912, 84.55) centre (-221.3313, 84.55) ccw
  line L140 (-221.3313, 83.51) -> (-226.3313, 83.51)
  arc A155 (-227.3713, 84.55) -> (-226.3313, 83.51) centre (-226.3313, 84.55) ccw
  line L141 (-227.3713, 84.55) -> (-227.3713, 97.55)
  arc A156 (-226.3313, 98.59) -> (-227.3713, 97.55) centre (-226.3313, 97.55) ccw
  line L142 (-226.3313, 98.59) -> (-221.3313, 98.59)
  arc A157 (-220.2913, 97.55) -> (-221.3313, 98.59) centre (-221.3313, 97.55) ccw
  line L143 (-220.2912, 97.55) -> (-220.2912, 84.55)
  line L144 (-322.763, 20.325) -> (-305.887, 20.325)
  line L145 (-305.887, 20.325) -> (-305.887, 21.325)
  arc A158 (-304.887, 22.325) -> (-305.887, 21.325) centre (-304.887, 21.325) ccw
  line L146 (-304.887, 22.325) -> (-299.887, 22.325)
  arc A159 (-298.887, 21.325) -> (-299.887, 22.325) centre (-299.887, 21.325) ccw
  line L147 (-298.887, 21.325) -> (-298.887, 20.3375)
  line L148 (-298.887, 20.3375) -> (-298.8, 20.3375)
  arc A160 (-297.8, 19.3375) -> (-298.8, 20.3375) centre (-298.8, 19.3375) ccw
  line L149 (-297.8, 19.3375) -> (-297.8, 7.3375)
  arc A161 (-298.8, 6.3375) -> (-297.8, 7.3375) centre (-298.8, 7.3375) ccw
  line L150 (-298.8, 6.3375) -> (-329.85, 6.3375)
  arc A162 (-330.85, 7.3375) -> (-329.85, 6.3375) centre (-329.85, 7.3375) ccw
  line L151 (-330.85, 7.3375) -> (-330.85, 19.3375)
  arc A163 (-329.85, 20.3375) -> (-330.85, 19.3375) centre (-329.85, 19.3375) ccw
  line L152 (-329.85, 20.3375) -> (-329.763, 20.3375)
  line L153 (-329.763, 20.3375) -> (-329.763, 21.325)
  arc A164 (-328.763, 22.325) -> (-329.763, 21.325) centre (-328.763, 21.325) ccw
  line L154 (-328.763, 22.325) -> (-323.763, 22.325)
  arc A165 (-322.763, 21.325) -> (-323.763, 22.325) centre (-323.763, 21.325) ccw
  line L155 (-322.763, 21.325) -> (-322.763, 20.325)
  arc A166 (-185.5938, 83.5375) -> (-184.5938, 82.5375) centre (-184.5938, 83.5375) ccw
  line L156 (-185.5938, 83.5375) -> (-185.5938, 95.5375)
  arc A167 (-184.5938, 96.5375) -> (-185.5938, 95.5375) centre (-184.5938, 95.5375) ccw
  line L157 (-184.5938, 96.5375) -> (-167.8313, 96.55)
  arc A168 (-166.8313, 95.55) -> (-167.8313, 96.55) centre (-167.8313, 95.55) ccw
  line L158 (-166.8313, 95.55) -> (-166.8313, 83.55)
  arc A169 (-167.8313, 82.55) -> (-166.8313, 83.55) centre (-167.8313, 83.55) ccw
  line L159 (-167.8313, 82.55) -> (-184.5938, 82.5375)
  arc A170 (-132.0557, 84.5375) -> (-131.0557, 83.5375) centre (-131.0557, 84.5375) ccw
  line L160 (-132.0557, 84.5375) -> (-132.0557, 97.5375)
  arc A171 (-131.0557, 98.5375) -> (-132.0557, 97.5375) centre (-131.0557, 97.5375) ccw
  line L161 (-131.0557, 98.5375) -> (-121.3312, 98.55)
  arc A172 (-120.3313, 97.55) -> (-121.3312, 98.55) centre (-121.3312, 97.55) ccw
  line L162 (-120.3312, 97.55) -> (-120.3312, 84.55)
  arc A173 (-121.3312, 83.55) -> (-120.3312, 84.55) centre (-121.3312, 84.55) ccw
  line L163 (-121.3312, 83.55) -> (-131.0557, 83.5375)
  arc A174 (-71.2938, 45.45) -> (-70.2938, 44.45) centre (-70.2938, 45.45) ccw
  line L164 (-71.2938, 45.45) -> (-71.2938, 57.45)
  arc A175 (-70.2938, 58.45) -> (-71.2938, 57.45) centre (-70.2938, 57.45) ccw
  line L165 (-70.2938, 58.45) -> (-53.5312, 58.4375)
  arc A176 (-52.5312, 57.4375) -> (-53.5312, 58.4375) centre (-53.5312, 57.4375) ccw
  line L166 (-52.5313, 57.4375) -> (-52.5313, 45.4375)
  arc A177 (-53.5312, 44.4375) -> (-52.5312, 45.4375) centre (-53.5312, 45.4375) ccw
  line L167 (-53.5312, 44.4375) -> (-70.2938, 44.45)
  arc A178 (-51.15, 6.3375) -> (-50.15, 7.3375) centre (-51.15, 7.3375) ccw
  line L168 (-51.15, 6.3375) -> (-63.15, 6.3375)
  arc A179 (-64.15, 7.3375) -> (-63.15, 6.3375) centre (-63.15, 7.3375) ccw
  line L169 (-64.15, 7.3375) -> (-64.15, 19.3375)
  arc A180 (-63.15, 20.3375) -> (-64.15, 19.3375) centre (-63.15, 19.3375) ccw
  line L170 (-63.15, 20.3375) -> (-51.15, 20.3375)
  arc A181 (-50.15, 19.3375) -> (-51.15, 20.3375) centre (-51.15, 19.3375) ccw
  line L171 (-50.15, 19.3375) -> (-50.15, 7.3375)
  arc A182 (-89.25, 6.3375) -> (-88.25, 7.3375) centre (-89.25, 7.3375) ccw
  line L172 (-89.25, 6.3375) -> (-101.25, 6.3375)
  arc A183 (-102.25, 7.3375) -> (-101.25, 6.3375) centre (-101.25, 7.3375) ccw
  line L173 (-102.25, 7.3375) -> (-102.25, 19.3375)
  arc A184 (-101.25, 20.3375) -> (-102.25, 19.3375) centre (-101.25, 19.3375) ccw
  line L174 (-101.25, 20.3375) -> (-89.25, 20.3375)
  arc A185 (-88.25, 19.3375) -> (-89.25, 20.3375) centre (-89.25, 19.3375) ccw
  line L175 (-88.25, 19.3375) -> (-88.25, 7.3375)
  arc A186 (-241.65, 6.3375) -> (-240.65, 7.3375) centre (-241.65, 7.3375) ccw
  line L176 (-241.65, 6.3375) -> (-253.65, 6.3375)
  arc A187 (-254.65, 7.3375) -> (-253.65, 6.3375) centre (-253.65, 7.3375) ccw
  line L177 (-254.65, 7.3375) -> (-254.65, 19.3375)
  arc A188 (-253.65, 20.3375) -> (-254.65, 19.3375) centre (-253.65, 19.3375) ccw
  line L178 (-253.65, 20.3375) -> (-241.65, 20.3375)
  arc A189 (-240.65, 19.3375) -> (-241.65, 20.3375) centre (-241.65, 19.3375) ccw
  line L179 (-240.65, 19.3375) -> (-240.65, 7.3375)
  arc A190 (-127.35, 6.3375) -> (-126.35, 7.3375) centre (-127.35, 7.3375) ccw
  line L180 (-127.35, 6.3375) -> (-139.35, 6.3375)
  arc A191 (-140.35, 7.3375) -> (-139.35, 6.3375) centre (-139.35, 7.3375) ccw
  line L181 (-140.35, 7.3375) -> (-140.35, 19.3375)
  arc A192 (-139.35, 20.3375) -> (-140.35, 19.3375) centre (-139.35, 19.3375) ccw
  line L182 (-139.35, 20.3375) -> (-127.35, 20.3375)
  arc A193 (-126.35, 19.3375) -> (-127.35, 20.3375) centre (-127.35, 19.3375) ccw
  line L183 (-126.35, 19.3375) -> (-126.35, 7.3375)
  arc A194 (-222.6, 6.3375) -> (-221.6, 7.3375) centre (-222.6, 7.3375) ccw
  line L184 (-222.6, 6.3375) -> (-234.6, 6.3375)
  arc A195 (-235.6, 7.3375) -> (-234.6, 6.3375) centre (-234.6, 7.3375) ccw
  line L185 (-235.6, 7.3375) -> (-235.6, 19.3375)
  arc A196 (-234.6, 20.3375) -> (-235.6, 19.3375) centre (-234.6, 19.3375) ccw
  line L186 (-234.6, 20.3375) -> (-222.6, 20.3375)
  arc A197 (-221.6, 19.3375) -> (-222.6, 20.3375) centre (-222.6, 19.3375) ccw
  line L187 (-221.6, 19.3375) -> (-221.6, 7.3375)
  arc A198 (-203.55, 6.3375) -> (-202.55, 7.3375) centre (-203.55, 7.3375) ccw
  line L188 (-203.55, 6.3375) -> (-215.55, 6.3375)
  arc A199 (-216.55, 7.3375) -> (-215.55, 6.3375) centre (-215.55, 7.3375) ccw
  line L189 (-216.55, 7.3375) -> (-216.55, 19.3375)
  arc A200 (-215.55, 20.3375) -> (-216.55, 19.3375) centre (-215.55, 19.3375) ccw
  line L190 (-215.55, 20.3375) -> (-203.55, 20.3375)
  arc A201 (-202.55, 19.3375) -> (-203.55, 20.3375) centre (-203.55, 19.3375) ccw
  line L191 (-202.55, 19.3375) -> (-202.55, 7.3375)
  arc A202 (-22.575, 6.3375) -> (-21.575, 7.3375) centre (-22.575, 7.3375) ccw
  line L192 (-22.575, 6.3375) -> (-34.575, 6.3375)
  arc A203 (-35.575, 7.3375) -> (-34.575, 6.3375) centre (-34.575, 7.3375) ccw
  line L193 (-35.575, 7.3375) -> (-35.575, 19.3375)
  arc A204 (-34.575, 20.3375) -> (-35.575, 19.3375) centre (-34.575, 19.3375) ccw
  line L194 (-34.575, 20.3375) -> (-22.575, 20.3375)
  arc A205 (-21.575, 19.3375) -> (-22.575, 20.3375) centre (-22.575, 19.3375) ccw
  line L195 (-21.575, 19.3375) -> (-21.575, 7.3375)
  arc A206 (-108.3, 6.3375) -> (-107.3, 7.3375) centre (-108.3, 7.3375) ccw
  line L196 (-108.3, 6.3375) -> (-120.3, 6.3375)
  arc A207 (-121.3, 7.3375) -> (-120.3, 6.3375) centre (-120.3, 7.3375) ccw
  line L197 (-121.3, 7.3375) -> (-121.3, 19.3375)
  arc A208 (-120.3, 20.3375) -> (-121.3, 19.3375) centre (-120.3, 19.3375) ccw
  line L198 (-120.3, 20.3375) -> (-108.3, 20.3375)
  arc A209 (-107.3, 19.3375) -> (-108.3, 20.3375) centre (-108.3, 19.3375) ccw
  line L199 (-107.3, 19.3375) -> (-107.3, 7.3375)
  arc A210 (-146.4, 6.3375) -> (-145.4, 7.3375) centre (-146.4, 7.3375) ccw
  line L200 (-146.4, 6.3375) -> (-158.4, 6.3375)
  arc A211 (-159.4, 7.3375) -> (-158.4, 6.3375) centre (-158.4, 7.3375) ccw
  line L201 (-159.4, 7.3375) -> (-159.4, 19.3375)
  arc A212 (-158.4, 20.3375) -> (-159.4, 19.3375) centre (-158.4, 19.3375) ccw
  line L202 (-158.4, 20.3375) -> (-146.4, 20.3375)
  arc A213 (-145.4, 19.3375) -> (-146.4, 20.3375) centre (-146.4, 19.3375) ccw
  line L203 (-145.4, 19.3375) -> (-145.4, 7.3375)
  arc A214 (-70.2, 6.3375) -> (-69.2, 7.3375) centre (-70.2, 7.3375) ccw
  line L204 (-70.2, 6.3375) -> (-82.2, 6.3375)
  arc A215 (-83.2, 7.3375) -> (-82.2, 6.3375) centre (-82.2, 7.3375) ccw
  line L205 (-83.2, 7.3375) -> (-83.2, 19.3375)
  arc A216 (-82.2, 20.3375) -> (-83.2, 19.3375) centre (-82.2, 19.3375) ccw
  line L206 (-82.2, 20.3375) -> (-70.2, 20.3375)
  arc A217 (-69.2, 19.3375) -> (-70.2, 20.3375) centre (-70.2, 19.3375) ccw
  line L207 (-69.2, 19.3375) -> (-69.2, 7.3375)
  arc A218 (-16.525, 7.3375) -> (-15.525, 6.3375) centre (-15.525, 7.3375) ccw
  line L208 (-16.525, 7.3375) -> (-16.525, 19.3375)
  arc A219 (-15.525, 20.3375) -> (-16.525, 19.3375) centre (-15.525, 19.3375) ccw
  line L209 (-15.525, 20.3375) -> (-3.525, 20.3375)
  arc A220 (-2.525, 19.3375) -> (-3.525, 20.3375) centre (-3.525, 19.3375) ccw
  line L210 (-2.525, 19.3375) -> (-2.525, 7.3375)
  arc A221 (-3.525, 6.3375) -> (-2.525, 7.3375) centre (-3.525, 7.3375) ccw
  line L211 (-3.525, 6.3375) -> (-15.525, 6.3375)
  arc A222 (-184.5, 6.3375) -> (-183.5, 7.3375) centre (-184.5, 7.3375) ccw
  line L212 (-184.5, 6.3375) -> (-196.5, 6.3375)
  arc A223 (-197.5, 7.3375) -> (-196.5, 6.3375) centre (-196.5, 7.3375) ccw
  line L213 (-197.5, 7.3375) -> (-197.5, 19.3375)
  arc A224 (-196.5, 20.3375) -> (-197.5, 19.3375) centre (-196.5, 19.3375) ccw
  line L214 (-196.5, 20.3375) -> (-184.5, 20.3375)
  arc A225 (-183.5, 19.3375) -> (-184.5, 20.3375) centre (-184.5, 19.3375) ccw
  line L215 (-183.5, 19.3375) -> (-183.5, 7.3375)
  arc A226 (-346.425, 87.3) -> (-345.425, 88.3) centre (-346.425, 88.3) ccw
  line L216 (-346.425, 87.3) -> (-358.425, 87.3)
  arc A227 (-359.425, 88.3) -> (-358.425, 87.3) centre (-358.425, 88.3) ccw
  line L217 (-359.425, 88.3) -> (-359.425, 100.3)
  arc A228 (-358.425, 101.3) -> (-359.425, 100.3) centre (-358.425, 100.3) ccw
  line L218 (-358.425, 101.3) -> (-346.425, 101.3)
  arc A229 (-345.425, 100.3) -> (-346.425, 101.3) centre (-346.425, 100.3) ccw
  line L219 (-345.425, 100.3) -> (-345.425, 88.3)
  arc A230 (-327.375, 87.3) -> (-326.375, 88.3) centre (-327.375, 88.3) ccw
  line L220 (-327.375, 87.3) -> (-339.375, 87.3)
  arc A231 (-340.375, 88.3) -> (-339.375, 87.3) centre (-339.375, 88.3) ccw
  line L221 (-340.375, 88.3) -> (-340.375, 100.3)
  arc A232 (-339.375, 101.3) -> (-340.375, 100.3) centre (-339.375, 100.3) ccw
  line L222 (-339.375, 101.3) -> (-327.375, 101.3)
  arc A233 (-326.375, 100.3) -> (-327.375, 101.3) centre (-327.375, 100.3) ccw
  line L223 (-326.375, 100.3) -> (-326.375, 88.3)
  arc A234 (-282.1313, 82.5375) -> (-281.1313, 83.5375) centre (-282.1313, 83.5375) ccw
  line L224 (-282.1313, 82.5375) -> (-294.1313, 82.5375)
  arc A235 (-295.1313, 83.5375) -> (-294.1313, 82.5375) centre (-294.1313, 83.5375) ccw
  line L225 (-295.1313, 83.5375) -> (-295.1313, 95.5375)
  arc A236 (-294.1313, 96.5375) -> (-295.1312, 95.5375) centre (-294.1313, 95.5375) ccw
  line L226 (-294.1313, 96.5375) -> (-282.1313, 96.5375)
  arc A237 (-281.1313, 95.5375) -> (-282.1313, 96.5375) centre (-282.1313, 95.5375) ccw
  line L227 (-281.1313, 95.5375) -> (-281.1313, 83.5375)
  arc A238 (-197.4932, 83.5375) -> (-196.4932, 84.5375) centre (-197.4932, 84.5375) ccw
  line L228 (-197.4932, 83.5375) -> (-202.4932, 83.5375)
  arc A239 (-203.4932, 84.5375) -> (-202.4932, 83.5375) centre (-202.4932, 84.5375) ccw
  line L229 (-203.4932, 84.5375) -> (-203.4932, 97.5375)
  arc A240 (-202.4932, 98.5375) -> (-203.4933, 97.5375) centre (-202.4933, 97.5375) ccw
  line L230 (-202.4932, 98.5375) -> (-197.4932, 98.5375)
  arc A241 (-196.4933, 97.5375) -> (-197.4932, 98.5375) centre (-197.4932, 97.5375) ccw
  line L231 (-196.4933, 97.5375) -> (-196.4932, 84.5375)
  arc A242 (-308.325, 87.3) -> (-307.325, 88.3) centre (-308.325, 88.3) ccw
  line L232 (-308.325, 87.3) -> (-320.325, 87.3)
  arc A243 (-321.325, 88.3) -> (-320.325, 87.3) centre (-320.325, 88.3) ccw
  line L233 (-321.325, 88.3) -> (-321.325, 100.3)
  arc A244 (-320.325, 101.3) -> (-321.325, 100.3) centre (-320.325, 100.3) ccw
  line L234 (-320.325, 101.3) -> (-308.325, 101.3)
  arc A245 (-307.325, 100.3) -> (-308.325, 101.3) centre (-308.325, 100.3) ccw
  line L235 (-307.325, 100.3) -> (-307.325, 88.3)
  arc A246 (-218.9313, 83.5375) -> (-217.9313, 82.5375) centre (-217.9313, 83.5375) ccw
  line L236 (-218.9313, 83.5375) -> (-218.9313, 95.5375)
  arc A247 (-217.9313, 96.5375) -> (-218.9313, 95.5375) centre (-217.9313, 95.5375) ccw
  line L237 (-217.9313, 96.5375) -> (-205.9313, 96.5375)
  arc A248 (-204.9313, 95.5375) -> (-205.9313, 96.5375) centre (-205.9312, 95.5375) ccw
  line L238 (-204.9313, 95.5375) -> (-204.9313, 83.5375)
  arc A249 (-205.9313, 82.5375) -> (-204.9312, 83.5375) centre (-205.9313, 83.5375) ccw
  line L239 (-205.9313, 82.5375) -> (-217.9313, 82.5375)
  arc A250 (-239.2688, 82.5375) -> (-238.2688, 83.5375) centre (-239.2688, 83.5375) ccw
  line L240 (-239.2688, 82.5375) -> (-251.2687, 82.5375)
  arc A251 (-252.2688, 83.5375) -> (-251.2688, 82.5375) centre (-251.2687, 83.5375) ccw
  line L241 (-252.2688, 83.5375) -> (-252.2687, 95.5375)
  arc A252 (-251.2687, 96.5375) -> (-252.2687, 95.5375) centre (-251.2687, 95.5375) ccw
  line L242 (-251.2687, 96.5375) -> (-239.2688, 96.5375)
  arc A253 (-238.2688, 95.5375) -> (-239.2688, 96.5375) centre (-239.2688, 95.5375) ccw
  line L243 (-238.2688, 95.5375) -> (-238.2688, 83.5375)
  arc A254 (-327.375, 68.25) -> (-326.375, 69.25) centre (-327.375, 69.25) ccw
  line L244 (-327.375, 68.25) -> (-339.375, 68.25)
  arc A255 (-340.375, 69.25) -> (-339.375, 68.25) centre (-339.375, 69.25) ccw
  line L245 (-340.375, 69.25) -> (-340.375, 81.25)
  arc A256 (-339.375, 82.25) -> (-340.375, 81.25) centre (-339.375, 81.25) ccw
  line L246 (-339.375, 82.25) -> (-327.375, 82.25)
  arc A257 (-326.375, 81.25) -> (-327.375, 82.25) centre (-327.375, 81.25) ccw
  line L247 (-326.375, 81.25) -> (-326.375, 69.25)
  arc A258 (-66.5312, 83.5375) -> (-65.5312, 82.5375) centre (-65.5312, 83.5375) ccw
  line L248 (-66.5312, 83.5375) -> (-66.5312, 95.5375)
  arc A259 (-65.5312, 96.5375) -> (-66.5313, 95.5375) centre (-65.5313, 95.5375) ccw
  line L249 (-65.5312, 96.5375) -> (-53.5312, 96.5375)
  arc A260 (-52.5313, 95.5375) -> (-53.5312, 96.5375) centre (-53.5312, 95.5375) ccw
  line L250 (-52.5313, 95.5375) -> (-52.5313, 83.5375)
  arc A261 (-53.5312, 82.5375) -> (-52.5312, 83.5375) centre (-53.5312, 83.5375) ccw
  line L251 (-53.5312, 82.5375) -> (-65.5312, 82.5375)
  arc A262 (-96.3938, 82.5375) -> (-95.3938, 83.5375) centre (-96.3938, 83.5375) ccw
  line L252 (-96.3938, 82.5375) -> (-108.3938, 82.5375)
  arc A263 (-109.3938, 83.5375) -> (-108.3938, 82.5375) centre (-108.3938, 83.5375) ccw
  line L253 (-109.3937, 83.5375) -> (-109.3937, 95.5375)
  arc A264 (-108.3938, 96.5375) -> (-109.3938, 95.5375) centre (-108.3938, 95.5375) ccw
  line L254 (-108.3938, 96.5375) -> (-96.3938, 96.5375)
  arc A265 (-95.3938, 95.5375) -> (-96.3938, 96.5375) centre (-96.3937, 95.5375) ccw
  line L255 (-95.3938, 95.5375) -> (-95.3938, 83.5375)
  arc A266 (-149.9318, 83.5375) -> (-148.9318, 84.5375) centre (-149.9317, 84.5375) ccw
  line L256 (-149.9318, 83.5375) -> (-154.9318, 83.5375)
  arc A267 (-155.9317, 84.5375) -> (-154.9318, 83.5375) centre (-154.9318, 84.5375) ccw
  line L257 (-155.9317, 84.5375) -> (-155.9317, 97.5375)
  arc A268 (-154.9317, 98.5375) -> (-155.9317, 97.5375) centre (-154.9318, 97.5375) ccw
  line L258 (-154.9318, 98.5375) -> (-149.9318, 98.5375)
  arc A269 (-148.9318, 97.5375) -> (-149.9317, 98.5375) centre (-149.9317, 97.5375) ccw
  line L259 (-148.9318, 97.5375) -> (-148.9318, 84.5375)
  line L260 (-21.575, 95.5375) -> (-21.575, 83.5375)
  arc A270 (-22.575, 82.5375) -> (-21.575, 83.5375) centre (-22.575, 83.5375) ccw
  line L261 (-22.575, 82.5375) -> (-34.575, 82.5375)
  arc A271 (-35.575, 83.5375) -> (-34.575, 82.5375) centre (-34.575, 83.5375) ccw
  line L262 (-35.575, 83.5375) -> (-35.575, 95.5375)
  arc A272 (-34.575, 96.5375) -> (-35.575, 95.5375) centre (-34.575, 95.5375) ccw
  line L263 (-34.575, 96.5375) -> (-22.575, 96.5375)
  arc A273 (-21.575, 95.5375) -> (-22.575, 96.5375) centre (-22.575, 95.5375) ccw
  arc A274 (-134.4938, 82.5375) -> (-133.4938, 83.5375) centre (-134.4938, 83.5375) ccw
  line L264 (-134.4938, 82.5375) -> (-146.4938, 82.5375)